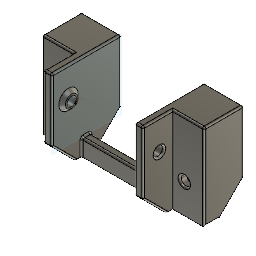
FoldingArm_2_Middle (Autodesk Fusion 360 design; units mm, degrees)
Autodesk Fusion 360 part; units mm, degrees
sketch "Sketch1" plane through (0, 0, 0) normal (0, 0, 1) x (1, 0, 0)
  line L0 (-25, 12.5) -> (-30, 12.5)
  line L1 (-30, 12.5) -> (-30, -12.5)
  line L2 (-30, -12.5) -> (-25, -12.5)
  line L3 (-25, -12.5) -> (-25, 12.5)
  line L4 (-49, 29.5) -> (-25, 29.5)
  line L5 (-25, 29.5) -> (-25, 5.5)
  line L6 (-25, 5.5) -> (-49, 5.5)
  line L7 (-49, 5.5) -> (-49, 29.5)
  line L8 (-30.2, 10.7) -> (-43.8, 10.7)
  line L9 (-43.8, 10.7) -> (-43.8, 24.3)
  line L10 (-43.8, 24.3) -> (-30.2, 24.3)
  line L11 (-30.2, 24.3) -> (-30.2, 10.7)
  line L12 (0, 1.75) -> (0, 22.5)
  line L13 (49, 5.5) -> (49, 29.5)
  line L14 (25, -12.5) -> (25, 12.5)
  line L15 (25, 29.5) -> (25, 5.5)
  line L16 (30.2, 10.7) -> (43.8, 10.7)
  line L17 (25, 5.5) -> (49, 5.5)
  line L18 (30, 12.5) -> (30, -12.5)
  line L19 (25, 12.5) -> (30, 12.5)
  line L20 (30.2, 24.3) -> (30.2, 10.7)
  line L21 (49, 29.5) -> (25, 29.5)
  line L22 (43.8, 10.7) -> (43.8, 24.3)
  line L23 (43.8, 24.3) -> (30.2, 24.3)
  line L24 (30, -12.5) -> (25, -12.5)
  dimension "d1" = 5
  dimension "d2" = 25
  dimension "d3" = 25
  dimension "d4" = 12.5
  dimension "d5" = 24
  dimension "d6" = 24
  dimension "d7" = 5.2
  dimension "d8" = 18
  constraint horizontal L0
  constraint vertical L1
  constraint horizontal L2
  constraint vertical L3
  constraint horizontal L4
  constraint vertical L5
  constraint horizontal L6
  constraint vertical L7
  constraint collinear L3 L5
  constraint symmetric L0.start L12 L14.end
  constraint symmetric L0.end L12 L18.start
  constraint symmetric L1.end L12 L18.end
  constraint symmetric L2.end L12 L14.start
  constraint symmetric L4.start L12 L13.end
  constraint symmetric L4.end L12 L15.start
  constraint symmetric L5.end L12 L15.end
  constraint symmetric L6.end L12 L13.start
  constraint symmetric L8.start L12 L16.start
  constraint symmetric L8.end L12 L16.end
  constraint symmetric L9.end L12 L22.end
  constraint symmetric L10.end L12 L20.start
  measures "d1" distance of L0.start L0.end
  measures "d2" distance of L0.start L2.end
  measures "d3" distance of origin L3
  measures "d4" vertical distance of origin L2.end
  measures "d5" distance of L4.start L4.end
  measures "d6" distance of L4.start L6.end
  measures "d8" distance of L2.end L6
extrude "Extrude1" add sketch "Sketch1" along normal blind 42 makes body 1 at (-25, 1.5, 14) makes body 2 at (25, 1.5, 14)
sketch "Sketch2" plane through (0, 0, 42) normal (0, 0, 1) x (-1, 0, 0)
  line L0 (-30.2, -24.3) -> (-43.8, -24.3)
  line L1 (-43.8, -24.3) -> (-43.8, -10.7)
  line L2 (-43.8, -10.7) -> (-30.2, -10.7)
  line L3 (-30.2, -10.7) -> (-30.2, -24.3)
  line L4 (-30, -5.5) -> (-49, -5.5)
  line L5 (-49, -5.5) -> (-49, -29.5)
  line L6 (-49, -29.5) -> (-25, -29.5)
  line L7 (-25, -29.5) -> (-25, 12.5)
  line L8 (-25, 12.5) -> (-30, 12.5)
  line L9 (-30, 12.5) -> (-30, -5.5)
  line L10 (49, -29.5) -> (49, -5.5)
  line L11 (43.8, -24.3) -> (30.2, -24.3)
  line L12 (30.2, -24.3) -> (30.2, -10.7)
  line L13 (30.2, -10.7) -> (43.8, -10.7)
  line L14 (43.8, -10.7) -> (43.8, -24.3)
  line L15 (30, -5.5) -> (30, 12.5)
  line L16 (30, 12.5) -> (25, 12.5)
  line L17 (25, 12.5) -> (25, -29.5)
  line L18 (25, -29.5) -> (49, -29.5)
  line L19 (49, -29.5) -> (49, -5.5)
  line L20 (49, -5.5) -> (30, -5.5)
extrude "Extrude2" add sketch "Sketch2" against normal blind 2.4 contours L0 L1 L2 L3 | L11 L12 L13 L14 bodies 1 2
sketch "Sketch3" plane through (0, 0, 0) normal (0, 0, -1) x (1, 0, 0)
  line L0 (43.8, -24.3) -> (30.2, -24.3)
  line L1 (30.2, -24.3) -> (30.2, -10.7)
  line L2 (30.2, -10.7) -> (43.8, -10.7)
  line L3 (43.8, -10.7) -> (43.8, -24.3)
  line L4 (49, -5.5) -> (30, -5.5)
  line L5 (30, -5.5) -> (30, 12.5)
  line L6 (30, 12.5) -> (25, 12.5)
  line L7 (25, 12.5) -> (25, -29.5)
  line L8 (25, -29.5) -> (49, -29.5)
  line L9 (49, -29.5) -> (49, -5.5)
  line L10 (49, -5.5) -> (-49, -5.5)
  line L11 (-49, -5.5) -> (-49, -10.7)
  line L12 (-49, -10.7) -> (49, -10.7)
  line L13 (49, -10.7) -> (49, -5.5)
  line L14 (-49, -5.5) -> (-49, -29.5)
  line L15 (-30.2, -10.7) -> (-43.8, -10.7)
  constraint horizontal L10
  constraint vertical L11
  constraint horizontal L12
  constraint vertical L13
  constraint coincident L4.start L9.end
  constraint collinear L11 L14
  constraint collinear L12 L15
extrude "Extrude3" add sketch "Sketch3" along normal blind 10 contours L2 L4 L7 L9 L10 L12 L13 | L7 L10 L11 L12 L14 L15 bodies 1 2
sketch "Sketch4" plane through (-30, 0, 0) normal (-1, 0, 0) x (0, -1, 0)
  line L0 (-5.5, 0) -> (12.5, 0)
  line L1 (12.5, 0) -> (12.5, 42)
  line L2 (12.5, 42) -> (-5.5, 42)
  line L3 (-5.5, 42) -> (-5.5, 0)
  circle A0 centre (2.5, 24) radius 2.8
  dimension "d15" = 5.6
  dimension "d16" = 10
  dimension "d17" = 18
  measures "d15" diameter of A0
  measures "d16" distance of L1 A0.centre
  measures "d17" distance of L2 A0.centre
extrude "Extrude4" cut sketch "Sketch4" against normal up to surface (60 mm away) contours A0 bodies 1
sketch "Sketch5" plane through (0, 29.5, 0) normal (0, 1, 0) x (-1, 0, 0)
  line L0 (25, 0) -> (49, 0)
  line L1 (49, 0) -> (49, 42)
  line L2 (49, 42) -> (25, 42)
  line L3 (25, 42) -> (25, 0)
  circle A0 centre (37, 8) radius 2.8
  line L4 (0, 1.75) -> (0, 22.5)
  circle A1 centre (-37, 8) radius 2.8
  dimension "d20" = 5.6
  dimension "d21" = 12
  dimension "d22" = 8
  constraint symmetric A0 L4 A1
  measures "d20" diameter of A0
  measures "d21" distance of L1 A0.centre
  measures "d22" distance of L0 A0.centre
extrude "Extrude5" cut sketch "Sketch5" against normal up to surface (24 mm away) contours A0 | A1 bodies 1
sketch "Sketch6" plane through (-25, 0, 0) normal (1, 0, 0) x (0, 1, 0)
  circle A0 centre (-2.5, 24) radius 2.8
  line L0 (-12.5, 0) -> (5.5, 0)
  line L1 (5.5, 0) -> (10.7, 0)
  line L2 (10.7, 0) -> (29.5, 0)
  line L3 (29.5, 0) -> (29.5, 42)
  line L4 (29.5, 42) -> (-12.5, 42)
  line L5 (-12.5, 42) -> (-12.5, 0)
sketch "Sketch7" plane through (-25, 0, 0) normal (1, 0, 0) x (0, 1, 0)
extrude "Extrude6" add 4 faces at (28.3333, -6.5, 0) (34.7333, 27.7667, 0) (-34.7333, 27.7667, 0) (-26.6667, -6.5, 0) along direction (0, 0, -1) up to surface end surface through (0, 0, -10) normal (0, 0, -1) offset 0 on bodies 1 bodies 1
chamfer "Chamfer2" distance 14 angle 45 4 edges at (27.5, -12.5, -10) (37, 29.5, -10) (-37, 29.5, -10) (-27.5, -12.5, -10) on bodies 1
sketch "Sketch8" plane through (25, 0, 0) normal (-1, 0, 0) x (0, -1, 0)
  circle A0 centre (2.5, 24) radius 2.8
  line L0 (-29.5, 4) -> (-15.5, -10)
  line L1 (-15.5, -10) -> (-10.7, -10)
  line L2 (-10.7, -10) -> (-10.7, 0)
  line L3 (-5.5, 0) -> (-5.5, -10)
  line L4 (-5.5, -10) -> (-1.5, -10)
  line L5 (-1.5, -10) -> (12.5, 4)
  line L6 (12.5, 4) -> (12.5, 42)
  line L7 (12.5, 42) -> (-29.5, 42)
  line L8 (-29.5, 42) -> (-29.5, 4)
  circle A1 centre (2.5, 24) radius 3.8
  line L9 (-10.7, 0) -> (-5.5, 0)
  dimension "d29" = 1
extrude "Extrude7" add sketch "Sketch8" along normal blind 2 contours A1 bodies 1
mirror "Mirror1" about plane through (0, 0, 0) normal (1, 0, 0) of "Extrude7"
chamfer "Chamfer4" distance 2 angle 45 2 edges at (25, 1.0428, 25.3741) (-25, 1.0428, 22.6259) on bodies 1
fillet "Fillet1" radius 1 6 edges at (-30, 0.1105, 25.0125) (30, 0.1105, 22.9875) (-25, 5.5, -5) (-25, 10.7, -5) (25, 5.5, -5) (25, 10.7, -5) 17 faces at (-39.7861, 7.2333, 7.7212) (34.2139, 8.9667, 7.7212) (34.2035, 26.0333, 7.8604) (34.6667, 21.5, 42) (-34.6667, 21.5, 42) (-39.7861, 26.0333, 7.7212) (-49, 13.5, 12) (-37.0697, 29.5, 31.5974) (36.9303, 29.5, 31.5974) (49, 13.5, 12) (-39.2667, 27.7667, 2.2667) (39.2667, 27.7667, 2.2667) (-28.3333, -3.1667, -5.3333) (28.3333, -3.1667, -5.3333) (28.3333, -12.5, 29.3333) (-28.3333, -12.5, 29.3333) (8.3333, 8.9667, 0) on bodies 1
named bodies: "FoldingArm_2_Middle"
